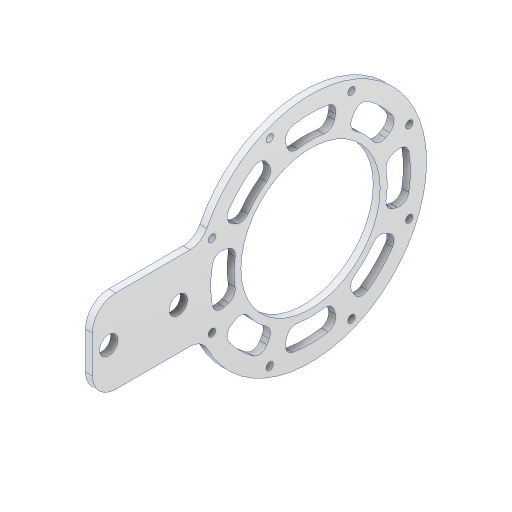
# Autodesk Inventor part: eobow_plate
Saved by Autodesk Inventor 2024.3 (Build 283343000, 343)
## iProperties
Created: 2024-10-12
Part Number: eobow_plate
Material: アルミニウム 6061
Document SubType Name: Sheet Metal
Designer: haya
Density: 2.7 g/cm^3
Sheet Metal Rule: plate_1_5
Appearance: アルミニウム - フラット
Mass: 47.1431 g
Surface Area: 153.115 cm^2
Volume: 17.4604 cm^3
Author: haya
Autodesk Inventor part; units mm, degrees
note: some values were not read from the file. Chosen so that the rebuilt part matches the saved one: direction of "穴2"; direction of "穴3"; direction of "穴4"; direction of "穴5"; direction of "穴6".
ref_plane "YZ Plane" through (0, 0, 0) normal (1, 0, 0) x (0, 1, 0)
ref_plane "XZ Plane" through (0, 0, 0) normal (0, 1, 0) x (-1, 0, 0)
ref_plane "XY Plane" through (0, 0, 0) normal (0, 0, 1) x (1, 0, 0)
sketch "スケッチ1" plane through (0, 0, 0) normal (0, 0, 1) x (1, 0, 0)
  line L0 (-20, 50) -> (20, 50)
  line L1 (20, 50) -> (20, -50)
  line L2 (20, -50) -> (-20, -50)
  line L3 (-20, -50) -> (-20, 50)
  line L4 (0, 0) -> (0, 50) construction
  line L5 (0, 0) -> (20, 0) construction
  dimension "d2" = 100
  dimension "d3" = 40
  measures "d2" distance of L0.end L1.end
  measures "d3" distance of L0.start L0.end
extrude "プレート1" add sketch "スケッチ1" along normal blind 3
sketch "スケッチ2" plane through (-23, 50, -3) normal (-1, 0, 0) x (0, -1, 0)
  line L0 (100, 0) -> (0, 0)
  line L1 (0, 0) -> (0, -102)
  line L2 (0, -102) -> (100, -102)
  line L3 (100, -102) -> (100, 0)
  constraints: 6 end point, 1 horizontal, 1 perpendicular, 1 vertical
edge flange "フランジ1" height 108 angle 90 thickness 3 bend radius 3 thickness toward (-1, 0, 0) relief tear relief width 3 relief depth 1.5 edges at (-20, 0, 0) wall of the first edge with corners at (-23, -50, -3) (-23, 50, -3) (-23, 50, -105) (-23, -50, -105)
bend "曲げ1"
corner "コーナー1"
sketch "スケッチ4" plane through (-26, -50, -105) normal (-1, 0, 0) x (0, 0, 1)
  line L0 (0, 100) -> (102, 100) projected
  line L1 (51, 100) -> (51, 0) construction
  line L2 (0, 0) -> (102, 0) projected
  line L3 (0, 0) -> (0, 100) projected
  line L4 (0, 50) -> (100, 50) construction
  circle A0 centre (50, 50) radius 50
  line L5 (51, 100) -> (0, 100)
  line L6 (0, 100) -> (0, 50)
  line L7 (0, 50) -> (0, 0)
  line L8 (0, 0) -> (51, 0)
  point P0 (105, 50)
  point P1 (0, 50)
  point P2 (50, 100)
  point P3 (50, 0)
  constraints: 12 end point, 4 midpoint, 3 collinear, 3 tangent, 1 centre point, 1 horizontal, 1 perpendicular
extrude "押し出し3" cut sketch "スケッチ4" against normal up to surface (3 mm away) contours L0 A0 L3 | A0 L2 L3
sketch "スケッチ6" plane through (0, 0, 3) normal (0, 0, 1) x (1, 0, 0)
  line L0 (20, -50) -> (20, 50) projected
  line L1 (20, 0) -> (-26, 0) construction
  line L2 (-26, 50) -> (-26, -50) projected
  point P0 (0, 0)
  point P1 (10.2, 0)
  point P2 (-5.1, 8.8335)
  point P3 (-5.1, -8.8335)
  dimension "d31" = 10.2
  dimension "d34" = 360
  dimension "d75" = 26
  constraints: 2 end point, 2 midpoint, 2 point on line, 4 other
  measures "d31" distance of point (10.2, 0) point (0, 0)
  measures "d75" distance from line of L2 point (0, 0)
hole "穴2" at (-5.1, 8.8335, 3) at (-5.1, -8.8335, 3) at (10.2, 0, 3) direction (0, 0, -1) diameter 4 depth 3
sketch "スケッチ7" plane through (0, 0, 3) normal (0, 0, 1) x (1, 0, 0)
  line L0 (20, -50) -> (20, 50) projected
  line L1 (20, 0) -> (-20, 0) construction
  line L2 (-20, 50) -> (-20, -50) projected
  line L3 (-26, -50) -> (-26, 50) projected
  point P0 (0, 0)
  point P1 (0, -12.5)
  point P2 (10.8253, -6.25)
  point P3 (10.8253, 6.25)
  point P4 (0, 12.5)
  point P5 (-10.8253, 6.25)
  point P6 (-10.8253, -6.25)
  dimension "d43" = 12.5
  dimension "d46" = 360
  dimension "d76" = 26
  constraints: 3 midpoint, 2 end point, 1 vertical alignment, 7 other
  measures "d43" distance of point (0, -12.5) point (0, 0)
  measures "d76" distance from line of point (0, 0) L3
hole "穴3" at (0, -12.5, 3) at (10.8253, -6.25, 3) at (10.8253, 6.25, 3) at (0, 12.5, 3) at (-10.8253, 6.25, 3) at (-10.8253, -6.25, 3) direction (0, 0, -1) diameter 3.2 depth 3
sketch "スケッチ8" plane through (-26, -50, -3) normal (-1, 0, 0) x (0, 0, 1)
  line L0 (-52, 100) -> (0, 100) projected
  arc A0 (-52, 100) -> (-52, 0) centre (-52, 50) ccw projected
  line L1 (-52, 100) -> (-52, 0) construction
  point P0 (3, 50)
  constraints: 2 end point, 1 vertical
hole "穴4" at (-26, 0, -55) direction (1, 0, 0) diameter 60 depth 3
sketch "スケッチ9" plane through (-26, -50, -3) normal (-1, 0, 0) x (0, 0, 1)
  arc A0 (-52, 100) -> (-52, 0) centre (-52, 50) ccw projected
  line L0 (-102, 50) -> (-52, 50) construction
  line L1 (-52, 50) -> (-98.194, 69.1342) construction
  point P0 (3, 50)
  point P1 (-94.4985, 67.6034)
  point P2 (-94.4985, 32.3966)
  point P3 (-69.6034, 7.5015)
  point P4 (-34.3966, 7.5015)
  point P5 (-9.5015, 32.3966)
  point P6 (-9.5015, 67.6034)
  point P7 (-34.3966, 92.4985)
  point P8 (-69.6034, 92.4985)
  dimension "d62" = 22.5
  dimension "d63" = 46
  dimension "d66" = 360
  constraints: 4 end point, 2 point on circle, 1 horizontal, 1 point on line, 9 other
  measures "d62" angle of L1 L0
  measures "d63" distance of point (-94.498, 67.603) L0.end
hole "穴5" at (-26, 17.6034, -97.4985) at (-26, -17.6034, -97.4985) at (-26, -42.4985, -72.6034) at (-26, -42.4985, -37.3966) at (-26, -17.6034, -12.5015) at (-26, 17.6034, -12.5015) at (-26, 42.4985, -37.3966) at (-26, 42.4985, -72.6034) direction (1, 0, 0) diameter 3.2 depth 3
sketch "スケッチ10" plane through (-26, -50, -3) normal (-1, 0, 0) x (0, 0, 1)
  arc A0 (-52, 100) -> (-52, 0) centre (-52, 50) ccw projected
  line L0 (-52, 0) -> (-52, 100) construction
  arc A1 (-7.3052, 72.4138) -> (-7.3052, 27.5862) centre (-52, 50) ccw
  line L1 (6, 100) -> (6, 0) projected
  line L2 (6, 32) -> (-0.1541, 32)
  line L3 (-52, 50) -> (6, 50) construction
  line L4 (6, 68) -> (-0.1541, 68)
  arc A2 (-0.1541, 32) -> (-7.3052, 27.5862) centre (-0.1541, 24) ccw
  arc A3 (-7.3052, 72.4138) -> (-0.1541, 68) centre (-0.1541, 76) ccw
  line L5 (-52, 0) -> (6, 0)
  line L6 (6, 100) -> (-52, 100)
  line L7 (6, 0) -> (6, 100)
  point P0 (3, 50)
  point P1 (-5.3524, 32)
  point P2 (-5.3524, 68)
  point P3 (6, 68)
  point P4 (-52, 0)
  dimension "d77" = 36
  dimension "d78" = 8
  dimension "d79" = 8
  constraints: 14 end point, 10 point on circle, 5 tangent, 3 centre point, 3 point on line, 2 symmetric about line, 1 coincident, 1 horizontal, 1 midpoint, 1 parallel, 1 perpendicular, 1 vertical
  measures "d77" distance between parallel lines of L4 L2
  measures "d78" radius of A2
  measures "d79" radius of A3
extrude "押し出し4" cut sketch "スケッチ10" against normal up to surface (46 mm away) contours L6 L1 L4 A3 A1 | A1 A2 L2 L1 L5
fillet "フィレット1" radius 10 2 edges at (20, -18, 1.5) (20, 18, 1.5)
sketch "スケッチ11" plane through (-26, 0, -55) normal (-1, 0, 0) x (0, 0, 1)
  arc A0 (-32.5191, 5.6134) -> (-32.5025, -5.7085) centre (0, 0) ccw
  circle A1 centre (0, 0) radius 30 projected
  arc A2 (-42.3319, 7.5505) -> (-42.3177, -7.6298) centre (0, 0) ccw
  arc A3 (44.6948, 22.4138) -> (44.6948, -22.4138) centre (0, 0) ccw projected
  line L0 (0, 0) -> (-37.2915, 10.6932) construction
  line L1 (0, 0) -> (-43, 0) construction
  line L2 (-35.4069, -10.2642) -> (-37.3459, -10.7837)
  arc A4 (-42.3177, -7.6298) -> (-37.3459, -10.7837) centre (-38.3812, -6.92) ccw
  arc A5 (-35.4069, -10.2642) -> (-32.5025, -5.7085) centre (-36.4422, -6.4005) ccw
  arc A6 (-32.5191, 5.6134) -> (-35.3582, 10.1388) centre (-36.4608, 6.2938) ccw
  arc A7 (-37.2915, 10.6932) -> (-42.3319, 7.5505) centre (-38.3941, 6.8481) ccw
  line L3 (-37.2915, 10.6932) -> (-35.3582, 10.1388)
  arc A8 (-33.9303, -18.8079) -> (-35.2722, -24.5942) centre (-31.991, -22.3063) ccw
  line L4 (-17.7786, -32.2943) -> (-18.7823, -34.0328)
  arc A9 (-35.2722, -24.5942) -> (-24.5281, -35.3182) centre (0, 0) ccw
  arc A10 (-24.5281, -35.3182) -> (-18.7823, -34.0328) centre (-22.2464, -32.0328) ccw
  arc A11 (-26.9637, -19.0252) -> (-18.9462, -27.0193) centre (0, 0) ccw
  line L5 (-33.9303, -18.8079) -> (-32.1713, -17.8328)
  arc A12 (-26.9637, -19.0252) -> (-32.1713, -17.8328) centre (-30.232, -21.3313) ccw
  arc A13 (-17.7786, -32.2943) -> (-18.9462, -27.0193) centre (-21.2427, -30.2943) ccw
  arc A14 (-10.6932, -37.2915) -> (-7.5505, -42.3319) centre (-6.8481, -38.3941) ccw
  line L6 (10.2642, -35.4069) -> (10.7837, -37.3459)
  arc A15 (-7.5505, -42.3319) -> (7.6298, -42.3177) centre (0, 0) ccw
  arc A16 (7.6298, -42.3177) -> (10.7837, -37.3459) centre (6.92, -38.3812) ccw
  arc A17 (-5.6134, -32.5191) -> (5.7085, -32.5025) centre (0, 0) ccw
  line L7 (-10.6932, -37.2915) -> (-10.1388, -35.3582)
  arc A18 (-5.6134, -32.5191) -> (-10.1388, -35.3582) centre (-6.2938, -36.4608) ccw
  arc A19 (10.2642, -35.4069) -> (5.7085, -32.5025) centre (6.4005, -36.4422) ccw
  arc A20 (18.8079, -33.9303) -> (24.5942, -35.2722) centre (22.3063, -31.991) ccw
  line L8 (32.2943, -17.7786) -> (34.0328, -18.7823)
  arc A21 (24.5942, -35.2722) -> (35.3182, -24.5281) centre (0, 0) ccw
  arc A22 (35.3182, -24.5281) -> (34.0328, -18.7823) centre (32.0328, -22.2464) ccw
  arc A23 (19.0252, -26.9637) -> (27.0193, -18.9462) centre (0, 0) ccw
  line L9 (18.8079, -33.9303) -> (17.8328, -32.1713)
  arc A24 (19.0252, -26.9637) -> (17.8328, -32.1713) centre (21.3313, -30.232) ccw
  arc A25 (32.2943, -17.7786) -> (27.0193, -18.9462) centre (30.2943, -21.2427) ccw
  arc A26 (37.2915, -10.6932) -> (42.3319, -7.5505) centre (38.3941, -6.8481) ccw
  line L10 (35.4069, 10.2642) -> (37.3459, 10.7837)
  arc A27 (42.3319, -7.5505) -> (42.3177, 7.6298) centre (0, 0) ccw
  arc A28 (42.3177, 7.6298) -> (37.3459, 10.7837) centre (38.3812, 6.92) ccw
  arc A29 (32.5191, -5.6134) -> (32.5025, 5.7085) centre (0, 0) ccw
  line L11 (37.2915, -10.6932) -> (35.3582, -10.1388)
  arc A30 (32.5191, -5.6134) -> (35.3582, -10.1388) centre (36.4608, -6.2938) ccw
  arc A31 (35.4069, 10.2642) -> (32.5025, 5.7085) centre (36.4422, 6.4005) ccw
  arc A32 (33.9303, 18.8079) -> (35.2722, 24.5942) centre (31.991, 22.3063) ccw
  line L12 (17.7786, 32.2943) -> (18.7823, 34.0328)
  arc A33 (35.2722, 24.5942) -> (24.5281, 35.3182) centre (0, 0) ccw
  arc A34 (24.5281, 35.3182) -> (18.7823, 34.0328) centre (22.2464, 32.0328) ccw
  arc A35 (26.9637, 19.0252) -> (18.9462, 27.0193) centre (0, 0) ccw
  line L13 (33.9303, 18.8079) -> (32.1713, 17.8328)
  arc A36 (26.9637, 19.0252) -> (32.1713, 17.8328) centre (30.232, 21.3313) ccw
  arc A37 (17.7786, 32.2943) -> (18.9462, 27.0193) centre (21.2427, 30.2943) ccw
  arc A38 (10.6932, 37.2915) -> (7.5505, 42.3319) centre (6.8481, 38.3941) ccw
  line L14 (-10.2642, 35.4069) -> (-10.7837, 37.3459)
  arc A39 (7.5505, 42.3319) -> (-7.6298, 42.3177) centre (0, 0) ccw
  arc A40 (-7.6298, 42.3177) -> (-10.7837, 37.3459) centre (-6.92, 38.3812) ccw
  arc A41 (5.6134, 32.5191) -> (-5.7085, 32.5025) centre (0, 0) ccw
  line L15 (10.6932, 37.2915) -> (10.1388, 35.3582)
  arc A42 (5.6134, 32.5191) -> (10.1388, 35.3582) centre (6.2938, 36.4608) ccw
  arc A43 (-10.2642, 35.4069) -> (-5.7085, 32.5025) centre (-6.4005, 36.4422) ccw
  arc A44 (-18.8079, 33.9303) -> (-24.5942, 35.2722) centre (-22.3063, 31.991) ccw
  line L16 (-32.2943, 17.7786) -> (-34.0328, 18.7823)
  arc A45 (-24.5942, 35.2722) -> (-35.3182, 24.5281) centre (0, 0) ccw
  arc A46 (-35.3182, 24.5281) -> (-34.0328, 18.7823) centre (-32.0328, 22.2464) ccw
  arc A47 (-19.0252, 26.9637) -> (-27.0193, 18.9462) centre (0, 0) ccw
  line L17 (-18.8079, 33.9303) -> (-17.8328, 32.1713)
  arc A48 (-19.0252, 26.9637) -> (-17.8328, 32.1713) centre (-21.3313, 30.232) ccw
  arc A49 (-32.2943, 17.7786) -> (-27.0193, 18.9462) centre (-30.2943, 21.2427) ccw
  point P0 (55, 0)
  point P1 (-41.3343, 11.8524)
  point P2 (-41.3343, -11.8524)
  point P3 (-31.6731, -9.2637)
  point P4 (-31.7216, 9.096)
  point P5 (-30.4056, -30.4056)
  point P6 (-20.8468, -37.6086)
  point P7 (-37.6086, -20.8468)
  point P8 (-28.8625, -15.9987)
  point P9 (-15.8458, -28.9467)
  point P10 (0, -43)
  point P11 (11.8524, -41.3343)
  point P12 (-11.8524, -41.3343)
  point P13 (-9.096, -31.7216)
  point P14 (9.2637, -31.6731)
  point P15 (30.4056, -30.4056)
  point P16 (37.6086, -20.8468)
  point P17 (20.8468, -37.6086)
  point P18 (15.9987, -28.8625)
  point P19 (28.9467, -15.8458)
  point P20 (43, 0)
  point P21 (41.3343, 11.8524)
  point P22 (41.3343, -11.8524)
  point P23 (31.7216, -9.096)
  point P24 (31.6731, 9.2637)
  point P25 (30.4056, 30.4056)
  point P26 (20.8468, 37.6086)
  point P27 (37.6086, 20.8468)
  point P28 (28.8625, 15.9987)
  point P29 (15.8458, 28.9467)
  point P30 (0, 43)
  point P31 (-11.8524, 41.3343)
  point P32 (11.8524, 41.3343)
  point P33 (9.096, 31.7216)
  point P34 (-9.2637, 31.6731)
  point P35 (-30.4056, 30.4056)
  point P36 (-37.6086, 20.8468)
  point P37 (-20.8468, 37.6086)
  point P38 (-15.9987, 28.8625)
  point P39 (-28.9467, 15.8458)
  dimension "d86" = 3
  dimension "d88" = 16
  dimension "d89" = 4
  dimension "d90" = 10
  dimension "d93" = 360
  constraints: 136 point on circle, 48 centre point, 36 end point, 20 point on line, 8 tangent, 3 coincident, 3 equal radius, 1 horizontal, 1 symmetric about line, 215 other
  measures "d86" radial gap between concentric circles of A0 A1
  measures "d88" angle of L1 L0
  measures "d89" radius of A4
  measures "d90" radial gap between concentric circles of A2 A0
extrude "押し出し5" cut sketch "スケッチ11" against normal up to surface (3 mm away) contours A0 A5 L2 A4 A2 A7 L3 A6 | L5 A12 A11 A13 L4 A10 A9 A8 | L7 A18 A17 A19 L6 A16 A15 A14 | L9 A24 A23 A25 L8 A22 A21 A20 | L11 A30 A29 A31 L10 A28 A27 A26 | L13 A36 A35 A37 L12 A34 A33 A32 | L15 A42 A41 A43 L14 A40 A39 A38 | L17 A48 A47 A49 L16 A46 A45 A44
sketch "スケッチ12" plane through (-26, 0, -55) normal (-1, 0, 0) x (0, 0, 1)
  line L0 (58, 18) -> (52, 18) projected
  line L1 (52, -18) -> (52, 18) projected
  line L2 (52, -18) -> (58, -18) projected
  line L3 (58, -18) -> (58, 18) projected
  point P0 (55, 0)
extrude "押し出し6" cut sketch "スケッチ12" against normal up to surface (46 mm away)
sketch "スケッチ13" plane through (-23, 0, -55) normal (1, 0, 0) x (0, 0, -1)
  line L0 (-52, -18) -> (-51.8459, -18) projected
  line L1 (-52, -18) -> (-94, -18)
  line L2 (-94, -18) -> (-94, 18)
  line L3 (-94, 18) -> (-52, 18)
  line L4 (-52, 18) -> (-52, -18)
  line L5 (-51.8459, 18) -> (-52, 18) projected
  point P0 (-55, 0)
  dimension "d99" = 42
  constraints: 8 end point, 2 parallel, 1 collinear, 1 horizontal, 1 perpendicular
  measures "d99" distance of L0.start L1.end
extrude "押し出し7" add sketch "スケッチ13" against normal up to surface (3 mm away)
sketch "スケッチ14" plane through (-23, 0, -55) normal (1, 0, 0) x (0, 0, -1)
  line L0 (-94, 18) -> (-94, -18) projected
  point P0 (-55, 0)
  point P1 (-57, 0)
  point P2 (-87, 0)
  dimension "d102" = 30
  dimension "d103" = 7
  measures "d102" distance of point (-87, 0) point (-57, 0)
  measures "d103" distance from line of point (-87, 0) L0
hole "穴6" at (-23, 0, 2) at (-23, 0, 32) direction (-1, 0, 0) diameter 7.9 depth 3
fillet "フィレット2" radius 10 2 edges at (-24.5, 18, 39) (-24.5, -18, 39)
equation "\"d109\" = Thickness"
equation "\"BendRadius\" = Thickness"
equation "\"BendReliefWidth\" = Thickness"
equation "\"BendReliefDepth\" = 0.5 * Thickness"
equation "\"CornerReliefSize\" = 4 * Thickness"
equation "\"MinimumRemnant\" = 2 * Thickness"
equation "\"TransitionRadius\" = BendRadius"
equation "\"JacobiRadiusSize\" = BendRadius"
equation "\"GapSize\" = Thickness"
